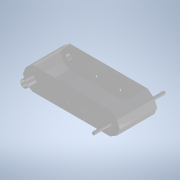
# Autodesk Inventor part: rama
Saved by Autodesk Inventor 2021 (Build 250183000, 183)
## iProperties
Created: 2021-06-23
Part Number: rama
Material: Generic
Document SubType Name: Modeling
Designer: Łukasz
Density: 1 g/cm^3
Appearance: Machined - Aluminum
Author: Łukasz
Autodesk Inventor part; units mm, degrees
ref_plane "YZ Plane" through (0, 0, 0) normal (1, 0, 0) x (0, 1, 0)
ref_plane "XZ Plane" through (0, 0, 0) normal (0, 1, 0) x (-1, 0, 0)
ref_plane "XY Plane" through (0, 0, 0) normal (0, 0, 1) x (1, 0, 0)
sketch "Sketch1" plane through (0, 0, 0) normal (0, 0, 1) x (1, 0, 0)
  circle A0 centre (0, 0) radius 14
  circle A1 centre (0, 0) radius 16
  dimension "d0" = 28
  dimension "d1" = 32
  constraints: 2 centre point, 2 coincident
  measures "d0" diameter of A0
  measures "d1" diameter of A1
extrude "Extrusion1" add sketch "Sketch1" along normal blind 35
sketch "Sketch3" plane through (0, 0, 35) normal (0, 0, 1) x (1, 0, 0)
  circle A0 centre (0, 0) radius 14
  arc A1 (-11.1364, -38.4185) -> (-20.0192, 34.6299) centre (0, 0) ccw construction
  line L0 (0, 0) -> (0, -45) construction
  line L1 (0, 0) -> (-28.2843, -28.2843) construction
  line L2 (0, 0) -> (40, 0) construction
  line L3 (-40, 0) -> (-28.2843, -28.2843)
  line L4 (-28.2843, -28.2843) -> (0, -45)
  line L5 (-40, 0) -> (10, 0) construction
  line L6 (0, -45) -> (162.5, -45)
  line L7 (0, 50) -> (162.5, 50)
  line L8 (162.5, 0) -> (162.5, -45) construction
  line L9 (0, 0) -> (0, 50) construction
  line L10 (0, 0) -> (-28.2843, 28.2843) construction
  line L11 (0, 0) -> (40, 0) construction
  line L12 (-40, 0) -> (-28.2843, 28.2843)
  line L13 (-28.2843, 28.2843) -> (0, 50)
  line L14 (325, 0) -> (325, -45) construction
  line L15 (325, 0) -> (285, 0) construction
  line L16 (325, 0) -> (325, 50) construction
  line L17 (325, 0) -> (285, 0) construction
  circle A2 centre (325, 0) radius 14
  arc A3 (345.0192, 34.6299) -> (336.1364, -38.4185) centre (325, 0) ccw construction
  line L18 (353.2843, 28.2843) -> (325, 50)
  line L19 (353.2843, -28.2843) -> (325, -45)
  line L20 (325, 0) -> (353.2843, 28.2843) construction
  line L21 (325, 0) -> (353.2843, -28.2843) construction
  line L22 (365, 0) -> (353.2843, 28.2843)
  line L23 (365, 0) -> (353.2843, -28.2843)
  line L24 (365, 0) -> (315, 0) construction
  line L25 (325, -45) -> (162.5, -45)
  line L26 (325, 50) -> (162.5, 50)
  dimension "d14" = 80
  dimension "d15" = 45
  dimension "d16" = 135
  dimension "d17" = 162.5
  dimension "d18" = 135
  dimension "d19" = 50
  constraints: 54 end point, 13 symmetric about line, 5 horizontal, 5 point on line, 4 centre point, 4 coincident, 4 point on circle, 2 equal length, 2 perpendicular, 1 vertical, 2 other
  measures "d14" diameter of A1
  measures "d15" distance of L0.start L6.start
  measures "d16" angle of L1 L2
  measures "d17" distance of L6.start L6.end
  measures "d18" angle of L11 L10
  measures "d19" distance from line of point (0, 0) L7
extrude "Extrusion3" add sketch "Sketch3" along normal blind 2 contours L12 L13 L7 L26 L18 L22 L23 L19 L25 L6 L4 L3 | A2
sketch "Sketch5" plane through (0, 0, 35) normal (0, 0, -1) x (-1, 0, 0)
  circle A0 centre (-325, 0) radius 6
  point P0 (0, 0)
  dimension "d22" = 12
  constraints: 2 coincident, 1 centre point
  measures "d22" diameter of A0
extrude "Extrusion4" add sketch "Sketch5" along normal blind 70
sketch "Sketch6" plane through (0, 0, 37) normal (0, 0, 1) x (1, 0, 0)
  line L0 (-28.2843, -28.2843) -> (0, -45) projected
  line L1 (0, -45) -> (325, -45) projected
  line L2 (325, -45) -> (353.2843, -28.2843) projected
  line L3 (353.2843, -28.2843) -> (365, 0) projected
  line L4 (365, 0) -> (353.2843, 28.2843) projected
  line L5 (353.2843, 28.2843) -> (325, 50) projected
  line L6 (325, 50) -> (0, 50) projected
  line L7 (0, 50) -> (-28.2843, 28.2843) projected
  line L8 (-28.2843, 28.2843) -> (-40, 0) projected
  line L9 (-40, 0) -> (-28.2843, -28.2843) projected
  circle A0 centre (0, 0) radius 14 projected
  line L10 (-26.6415, 27.0241) -> (0.6792, 48)
  line L11 (324.3208, 48) -> (351.6415, 27.0241)
  line L12 (351.6415, 27.0241) -> (362.8352, 0)
  line L13 (362.8352, 0) -> (351.692, -26.9021)
  line L14 (351.692, -26.9021) -> (324.4532, -43)
  line L15 (324.4532, -43) -> (0.5468, -43)
  line L16 (0.5468, -43) -> (-26.692, -26.9021)
  line L17 (-26.692, -26.9021) -> (-37.8352, 0)
  line L18 (-37.8352, 0) -> (-26.6415, 27.0241)
  line L19 (0, 50) -> (-28.2843, 28.2843) projected
  line L20 (0, 50) -> (0, 47.4785)
  line L21 (324.3208, 48) -> (324.3208, 50)
  line L22 (325, 50) -> (0, 50) projected
  dimension "d25" = 2
  constraints: 22 end point, 2 point on line, 1 perpendicular, 1 vertical, 7 other
  measures "d25" distance between parallel lines of L7 L10
extrude "Extrusion5" add sketch "Sketch6" along normal blind 152.8 contours L9 L8 L7 L20 L10 L18 L17 L16 L15 L14 L13 L12 L11 L21 L6 L5 L4 L3 L2 L1 L0
sketch "Sketch7" plane through (0, 0, 189.8) normal (0, 0, 1) x (1, 0, 0)
  circle A0 centre (0, 0) radius 14 projected
  line L0 (0, 50) -> (0, 47.4785) projected
  line L1 (0, 47.4785) -> (-26.6415, 27.0241) projected
  line L2 (-26.6415, 27.0241) -> (-37.8352, 0) projected
  line L3 (-37.8352, 0) -> (-26.692, -26.9021) projected
  line L4 (-26.692, -26.9021) -> (0.5468, -43) projected
  line L5 (0.5468, -43) -> (324.4532, -43) projected
  line L6 (324.4532, -43) -> (351.692, -26.9021) projected
  line L7 (351.692, -26.9021) -> (362.8352, 0) projected
  line L8 (362.8352, 0) -> (351.6415, 27.0241) projected
  line L9 (351.6415, 27.0241) -> (324.3208, 48) projected
  line L10 (324.3208, 48) -> (324.3208, 50) projected
  line L11 (324.3208, 50) -> (0, 50) projected
  line L12 (325, 50) -> (324.3208, 50) projected
  line L13 (324.3208, 50) -> (324.3208, 48) projected
  line L14 (324.3208, 48) -> (351.6415, 27.0241) projected
  line L15 (351.6415, 27.0241) -> (362.8352, 0) projected
  line L16 (362.8352, 0) -> (351.692, -26.9021) projected
  line L17 (351.692, -26.9021) -> (324.4532, -43) projected
  line L18 (324.4532, -43) -> (0.5468, -43) projected
  line L19 (0.5468, -43) -> (-26.692, -26.9021) projected
  line L20 (-26.692, -26.9021) -> (-37.8352, 0) projected
  line L21 (-37.8352, 0) -> (-26.6415, 27.0241) projected
  line L22 (-26.6415, 27.0241) -> (0, 47.4785) projected
  line L23 (0, 47.4785) -> (0, 50) projected
  line L24 (0, 50) -> (-28.2843, 28.2843) projected
  line L25 (-28.2843, 28.2843) -> (-40, 0) projected
  line L26 (-40, 0) -> (-28.2843, -28.2843) projected
  line L27 (-28.2843, -28.2843) -> (0, -45) projected
  line L28 (0, -45) -> (325, -45) projected
  line L29 (325, -45) -> (353.2843, -28.2843) projected
  line L30 (353.2843, -28.2843) -> (365, 0) projected
  line L31 (365, 0) -> (353.2843, 28.2843) projected
  line L32 (353.2843, 28.2843) -> (325, 50) projected
extrude "Extrusion6" add sketch "Sketch7" along normal blind 2
sketch "Sketch8" plane through (0, 0, 191.8) normal (0, 0, 1) x (1, 0, 0)
  circle A0 centre (0, 0) radius 14 projected
  circle A1 centre (0, 0) radius 16 projected
extrude "Extrusion7" add sketch "Sketch8" along normal blind 35
sketch "Sketch9" plane through (0, 0, 191.8) normal (0, 0, 1) x (1, 0, 0)
  circle A0 centre (325, 0) radius 6 projected
  point P0 (0, 0)
extrude "Extrusion8" add sketch "Sketch9" along normal blind 70
sketch "Sketch12" plane through (0, 0, 191.8) normal (0, 0, 1) x (1, 0, 0)
  circle A0 centre (147.5, -11.5574) radius 4 projected
  circle A1 centre (177.5, -11.5574) radius 4 projected
  point P0 (0, 0)
extrude "Extrusion11" cut sketch "Sketch12" against normal up to surface (2 mm away)
sketch "Sketch13" plane through (0, 0, 37) normal (0, 0, 1) x (1, 0, 0)
  circle A0 centre (147.5, -11.5574) radius 4 projected
  circle A1 centre (177.5, -11.5574) radius 4 projected
  point P0 (0, 0)
extrude "Extrusion12" cut sketch "Sketch13" against normal up to surface (2 mm away)
body "Solid1"
